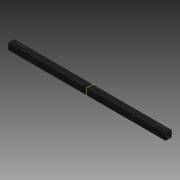
# Autodesk Inventor part: KozepsoOsszekotok
Saved by Autodesk Inventor 2015 (Build 190159000, 159)
## iProperties
Created: 2014-09-27
Part Number: KozepsoOsszekotok
Material: Steel, Alloy
Document SubType Name: Modeling
Designer: laca
Density: 7.73 g/cm^3
Appearance: Semi-Polished
Mass: 236.108 g
Surface Area: 410.763 cm^2
Volume: 30.5444 cm^3
Author: laca
Autodesk Inventor part; units mm, degrees
ref_plane "YZ Plane" through (0, 0, 0) normal (1, 0, 0) x (0, 1, 0)
ref_plane "XZ Plane" through (0, 0, 0) normal (0, 1, 0) x (-1, 0, 0)
ref_plane "XY Plane" through (0, 0, 0) normal (0, 0, 1) x (1, 0, 0)
derived "KétvégenMartSzelvény.ipt"
sketch "Sketch1" plane through (0, 0, 0) normal (1, 0, 0) x (0, 1, 0)
  line L0 (0, 0) -> (12, 0)
  line L1 (12, 0) -> (12, 12)
  line L2 (12, 12) -> (0, 12)
  line L3 (0, 12) -> (0, 0)
  line L4 (-1.5, 13.5) -> (13.5, 13.5)
  line L5 (13.5, 13.5) -> (13.5, -1.5)
  line L6 (13.5, -1.5) -> (-1.5, -1.5)
  line L7 (-1.5, -1.5) -> (-1.5, 13.5)
extrude "Extrusion1" add sketch "Sketch1" along normal blind 380
sketch "Sketch3" plane through (0, -1.5, -1.5) normal (0, -1, 0) x (1, 0, 0)
  arc A0 (13.094, 10) -> (13.094, 5) centre (13.094, 7.5) ccw
  arc A1 (28.094, 5) -> (28.094, 10) centre (28.094, 7.5) ccw
  line L0 (0, 15) -> (380, 15) projected
  line L1 (0, 0) -> (380, 0) projected
  line L2 (0, 0) -> (0, 15) projected
  line L3 (13.094, 10) -> (28.094, 10)
  line L4 (13.094, 5) -> (28.094, 5)
  point P0 (0, 1.5)
  dimension "d7" = 5
  dimension "d10" = 5
  dimension "d11" = 7.5
  dimension "d14" = 15
  dimension "d16" = 7.5
  dimension "d17" = 15
  dimension "d18" = 13.094
  constraints: 4 end point, 4 point on circle, 2 centre point, 2 tangent, 1 horizontal
  measures "d7" diameter of A0
  measures "d10" diameter of A1
  measures "d11" distance from line of L0 A0.centre
  measures "d14" distance between parallel lines of L1 L0
  measures "d16" distance from line of L0 A1.centre
  measures "d17" distance of A1.centre A0.centre
  measures "d18" distance from line of L2 A0.centre
extrude "Extrusion2" cut sketch "Sketch3" against normal through all
ref_plane "Work Plane1" through (190, -1.5, 13.5) normal (-1, 0, 0) x (0, 0, 1)
mirror "Mirror1" about plane through (190, -1.5, 13.5) normal (-1, 0, 0) of "Extrusion2"
equation "\"d11\" = 0.5 * d14"
equation "\"d16\" = d11"
body "Solid1"
